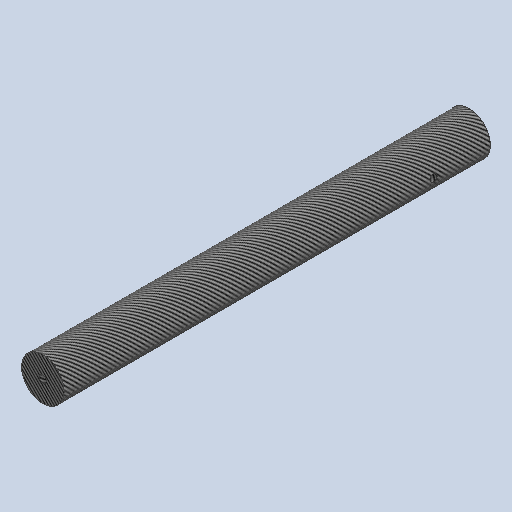
# Autodesk Inventor part: Shaft connecting chass
Saved by Autodesk Inventor 2023 (Build 270158000, 158)
## iProperties
Created: 2022-01-19
Part Number: Shaft connecting chass
Material: CFRP
Document SubType Name: Modeling
Designer: raymo
Density: 1.43 g/cm^3
Appearance: Carbon Fiber
Author: raymo
Autodesk Inventor part; units mm, degrees
ref_plane "YZ Plane" through (0, 0, 0) normal (1, 0, 0) x (0, 1, 0)
ref_plane "XZ Plane" through (0, 0, 0) normal (0, 1, 0) x (-1, 0, 0)
ref_plane "XY Plane" through (0, 0, 0) normal (0, 0, 1) x (1, 0, 0)
sketch "Sketch6" plane through (0, 0, 0) normal (0, 0, 1) x (1, 0, 0)
  circle A0 centre (0, 0) radius 3.175
  circle A1 centre (0, 0) radius 19.05
  dimension "d17" = 6.35
  dimension "d18" = 38.1
  constraints: 2 centre point, 2 coincident
  measures "d17" diameter of A0
  measures "d18" diameter of A1
extrude "Extrusion5" add sketch "Sketch6" along normal blind 381
sketch "Sketch7" plane through (0, 0, 0) normal (1, 0, 0) x (0, 1, 0)
  circle A0 centre (0, 50.8) radius 3.175
  line L0 (19.05, 0) -> (-19.05, 0) projected
  line L1 (19.05, 0) -> (19.05, 27.0227)
  line L2 (19.05, 0) -> (19.05, 381) projected
  line L3 (-19.05, 0.4439) -> (-19.05, 5.396)
  line L4 (-19.05, 0) -> (-19.05, 381) projected
  point P0 (0, 0)
  point P1 (0, 0)
  dimension "d21" = 6.35
  dimension "d22" = 19.05
  dimension "d23" = 19.05
  dimension "d24" = 50.8
  constraints: 4 end point, 2 point on line, 1 centre point, 1 midpoint
  measures "d21" diameter of A0
  measures "d22" distance from line of L1 A0.centre
  measures "d23" distance from line of L3 A0.centre
  measures "d24" distance of point (0, 0) A0.centre
extrude "Extrusion6" cut sketch "Sketch7" along normal mid plane 127
body "Solid2"
